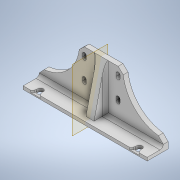
# Autodesk Inventor part: camera mount
Saved by Autodesk Inventor 2022.6 (Build 266554000, 554)
## iProperties
Created: 2024-11-11
Part Number: camera mount
Material: Generic
Document SubType Name: Modeling
Designer: Admin
Density: 1 g/cm^3
Appearance: Default
Author: Admin
Autodesk Inventor part; units mm, degrees
ref_plane "YZ Plane" through (0, 0, 0) normal (1, 0, 0) x (0, 1, 0)
ref_plane "XZ Plane" through (0, 0, 0) normal (0, 1, 0) x (-1, 0, 0)
ref_plane "XY Plane" through (0, 0, 0) normal (0, 0, 1) x (1, 0, 0)
sketch "Sketch1" plane through (0, 0, 0) normal (1, 0, 0) x (0, 1, 0)
  line L0 (0, 0) -> (2, 0)
  line L1 (2, 0) -> (2, 13)
  line L2 (2, 13) -> (0, 13)
  line L3 (0, 13) -> (0, 0)
  line L4 (0, 0) -> (32, 0)
  line L5 (32, 0) -> (32, 3)
  line L6 (32, 3) -> (0, 3)
  line L7 (0, 3) -> (0, 0)
  point P0 (2, 3)
  dimension "d0" = 32
  dimension "d1" = 2
  dimension "d2" = 13
  dimension "d3" = 3
  constraints: 16 end point, 4 parallel, 2 horizontal, 2 perpendicular
  measures "d0" distance of L5.end L6.end
  measures "d1" distance between parallel lines of L3 L1
  measures "d2" distance of L0.end L1.end
  measures "d3" distance of L4.end L5.end
extrude "Extrusion1" add sketch "Sketch1" along normal blind 77
sketch "Sketch2" plane through (0, 2, 13) normal (0, 1, 0) x (1, 0, 0)
  line L0 (0, 10) -> (0, 0) construction
  line L1 (0, 3) -> (77, 3) construction
  line L2 (0, 10) -> (0, 0) construction
  line L3 (0, 0) -> (77, 0) construction
  line L4 (77, 10) -> (77, 0) construction
  line L5 (0, 10) -> (77, 10) construction
  line L6 (77, 10) -> (77, 0) construction
  line L7 (0, 0) -> (77, 0) projected
  line L8 (38.5, 0) -> (38.5, 10)
  line L9 (0, 10) -> (77, 10) projected
  point P0 (0, 13)
  point P1 (7.75, 3)
  point P2 (69.25, 3)
  dimension "d6" = 3
  dimension "d7" = 61.5
  constraints: 4 end point, 4 point on line, 2 midpoint, 1 horizontal, 1 symmetric about line
  measures "d6" distance between parallel lines of L3 L1
  measures "d7" distance of point (7.75, 3) point (69.25, 3)
hole "Hole1" at (7.75, 2, 10) at (69.25, 2, 10) direction (0, -1, 0) diameter 3.4 end through all
ref_plane "Work Plane1" through (38.5, 0, 0) normal (1, 0, 0) x (0, 0, -1)
sketch "Sketch3" plane through (38.5, 0, 0) normal (1, 0, 0) x (0, 0, -1)
  line L0 (-3, 32) -> (-3, 2) projected
  line L1 (-3, 2) -> (-13, 2) projected
  line L2 (-13, 2) -> (-13, 0) projected
  line L3 (-13, 0) -> (0, 0) projected
  line L4 (0, 0) -> (0, 32) projected
  line L5 (0, 32) -> (-3, 32) projected
  line L6 (-3, 2) -> (-13, 2) projected
  line L7 (-10, 2) -> (-3, 32)
  line L8 (-3, 32) -> (-3, 2) projected
  dimension "d16" = 7
  dimension "d17" = 30
  constraints: 2 end point, 2 point on line
  measures "d16" distance from line of L0 L7.start
  measures "d17" distance from line of L1 L7.end
extrude "Rib1" add sketch "Sketch3" along normal mid plane 5 rib yes fills toward (-6.4513, 16.9886) open curves L7
sketch "Sketch4" plane through (0, 2, 3) normal (0, 0, 1) x (1, 0, 0)
  line L0 (36, 0) -> (36, 30) projected
  line L1 (41, 30) -> (41, 0) projected
  line L2 (41, 0) -> (77, 0) projected
  line L3 (77, 30) -> (77, 0) projected
  line L4 (0, 30) -> (36, 30) projected
  line L5 (0, 30) -> (0, 0) projected
  line L6 (0, 0) -> (36, 0) projected
  line L7 (0, 30) -> (77, 30) projected
  line L8 (0, 30) -> (0, 0) projected
  line L9 (38.5, 36.4) -> (38.5, -8.4) projected
  line L10 (0, -1) -> (0, 30)
  line L11 (25, 30) -> (0, 30)
  line L12 (77, -1) -> (77, 30)
  line L13 (52, 30) -> (77, 30)
  line L14 (41, 30) -> (77, 30) projected
  arc A0 (0, 5) -> (25, 30) centre (0, 30) ccw
  line L15 (0, 30) -> (77, 30) projected
  line L16 (0, 5) -> (0, 30)
  arc A1 (52, 30) -> (77, 5) centre (77, 30) ccw
  point P0 (0, -2)
  point P1 (77, 5)
  point P2 (0, 5)
  dimension "d24" = 25
  constraints: 10 end point, 4 point on circle, 4 symmetric about line, 3 point on line, 2 centre point, 2 collinear, 2 line through centre, 1 perpendicular, 1 other
  measures "d24" distance of L4.start L11.start
extrude "Extrusion2" cut sketch "Sketch4" against normal through all contours A0 L5 L4 | L7 L3 A1
sketch "Sketch5" plane through (77, 0, 0) normal (0, 0, -1) x (-1, 0, 0)
  line L0 (0, 0) -> (0, 7) projected
  line L1 (77, 0) -> (0, 0) projected
  line L2 (77, 0) -> (77, 7) projected
  line L3 (52, 32) -> (25, 32) projected
  line L4 (28, 26) -> (49, 26) construction
  line L5 (49, 26) -> (49, 13) construction
  line L6 (49, 13) -> (28, 13) construction
  line L7 (28, 13) -> (28, 26) construction
  line L8 (38.5, -7.4948) -> (38.5, 42.0825) construction
  line L9 (28, 26) -> (28, 27.8) construction
  line L10 (29.2, 26) -> (29.2, 27.8)
  line L11 (26.8, 27.8) -> (26.8, 26)
  arc A0 (26.8, 26) -> (29.2, 26) centre (28, 26) ccw
  arc A1 (29.2, 27.8) -> (26.8, 27.8) centre (28, 27.8) ccw
  line L12 (50.2, 26) -> (50.2, 27.8)
  line L13 (49, 26) -> (49, 27.8) construction
  line L14 (47.8, 27.8) -> (47.8, 26)
  arc A2 (47.8, 26) -> (50.2, 26) centre (49, 26) ccw
  arc A3 (50.2, 27.8) -> (47.8, 27.8) centre (49, 27.8) ccw
  line L15 (29.2, 13) -> (29.2, 14.8)
  line L16 (28, 13) -> (28, 14.8) construction
  line L17 (26.8, 14.8) -> (26.8, 13)
  arc A4 (26.8, 13) -> (29.2, 13) centre (28, 13) ccw
  arc A5 (29.2, 14.8) -> (26.8, 14.8) centre (28, 14.8) ccw
  line L18 (50.2, 13) -> (50.2, 14.8)
  line L19 (49, 13) -> (49, 14.8) construction
  line L20 (47.8, 14.8) -> (47.8, 13)
  arc A6 (47.8, 13) -> (50.2, 13) centre (49, 13) ccw
  arc A7 (50.2, 14.8) -> (47.8, 14.8) centre (49, 14.8) ccw
  arc A8 (0, 7) -> (25, 32) centre (0, 32) ccw projected
  arc A9 (52, 32) -> (77, 7) centre (77, 32) ccw projected
  point P0 (28, 26.9)
  point P1 (49, 26.9)
  point P2 (28, 13.9)
  point P3 (49, 13.9)
  dimension "d28" = 21
  dimension "d29" = 13
  dimension "d30" = 13
  dimension "d31" = 1.8
  dimension "d32" = 2.4
  dimension "d35" = 21
  dimension "d38" = 13
  constraints: 40 end point, 16 point on circle, 8 centre point, 4 tangent, 3 parallel, 2 horizontal, 2 vertical, 1 midpoint, 1 perpendicular, 37 other
  measures "d28" distance of L5.end L6.end
  measures "d29" distance of L4.end L5.end
  measures "d30" distance between parallel lines of L1 L6
  measures "d31" distance of L4.start L9.end
  measures "d32" diameter of A1
  measures "d35" distance of L10.end L12.end
  measures "d38" distance of L10.end L15.end
extrude "Cam holes" cut sketch "Sketch5" against normal through all contours A0 L11 A1 L10 | A2 L14 A3 L12 | A4 L17 A5 L15 | A6 L20 A7 L18
fillet "Fillet1" radius 2 4 edges at (59, 2, 3) (18, 2, 3) (41, 17, 3) (36, 17, 3)
sketch "Sketch6" plane through (0, 2, 13) normal (0, 1, 0) x (1, 0, 0)
  line L0 (0, 8) -> (36, 8) projected
  line L1 (0, 8) -> (0, 0) projected
  line L2 (0, 0) -> (77, 0) projected
  line L3 (41, 8) -> (41, 3) projected
  line L4 (41, 3) -> (36, 3) projected
  line L5 (36, 3) -> (36, 8) projected
  circle A0 centre (7.75, 3) radius 1.7 projected
  circle A1 centre (69.25, 3) radius 1.7 projected
  line L6 (7.75, 0) -> (7.75, 1) construction
  line L7 (5.75, 0) -> (5.75, 1)
  line L8 (9.75, 1) -> (9.75, 0)
  arc A2 (5.75, 0) -> (9.75, 0) centre (7.75, 0) ccw
  arc A3 (9.75, 1) -> (5.75, 1) centre (7.75, 1) ccw
  line L9 (0, 0) -> (77, 0) projected
  line L10 (38.5, 16) -> (38.5, -5) projected
  line L11 (77, 0) -> (0, 0)
  circle A4 centre (69.25, 3) radius 1.7
  line L12 (69.25, 0) -> (69.25, 1) construction
  line L13 (71.25, 0) -> (71.25, 1)
  line L14 (67.25, 1) -> (67.25, 0)
  arc A5 (67.25, 0) -> (71.25, 0) centre (69.25, 0) ccw
  arc A6 (71.25, 1) -> (67.25, 1) centre (69.25, 1) ccw
  line L15 (77, 0) -> (0, 0)
  line L16 (77, 8) -> (77, 0) projected
  line L17 (41, 8) -> (77, 8) projected
  point P0 (0, 13)
  point P1 (7.75, 0.5)
  point P2 (9.2888, 2.2775)
  point P3 (6.2112, 2.2775)
  point P4 (5.75, 0)
  point P5 (9.75, 0)
  point P6 (69.25, 0.5)
  point P7 (71.25, 0)
  point P8 (70.7888, 2.2775)
  point P9 (67.7112, 2.2775)
  point P10 (67.25, 0)
  dimension "d47" = 1
  dimension "d50" = 4
  constraints: 20 end point, 10 symmetric about line, 8 point on circle, 5 centre point, 4 tangent, 2 point on line, 2 vertical alignment, 1 midpoint, 1 parallel, 1 perpendicular, 3 other
  measures "d47" distance of L6.start L6.end
  measures "d50" distance between parallel lines of L8 L7
extrude "Extrusion4" cut sketch "Sketch6" against normal blind 1.3 contours L7 A3 A0 L8 L2 | L14 A6 A1 L13 L2
chamfer "Chamfer1" distance 1 angle 45 4 edges at (67.25, 1.35, 13) (71.25, 1.35, 13) (5.75, 1.35, 13) (9.75, 1.35, 13)
chamfer "Chamfer2" distance 3 angle 45 4 edges at (52, 32, 1.5) (25, 32, 1.5) (77, 7, 1.5) (0, 7, 1.5)
equation "\"d35\" = d28"
equation "\"d38\" = d29"
body "Solid1"
